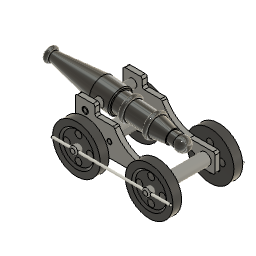
cannon v2 (Autodesk Fusion 360 design; units mm, degrees)
Autodesk Fusion 360 part; units mm, degrees
sketch "Sketch1" plane through (0, 0, 0) normal (0, 0, 1) x (1, 0, 0) in component "Component"
  line L0 (95, 0) -> (95, 20)
  line L1 (20, 50) -> (0, 50)
  line L2 (0, 50) -> (0, 0)
  line L3 (20, 50) -> (20, 40)
  line L4 (68.7228, 20) -> (95, 20)
  line L5 (75, 0) -> (75, 10)
  line L6 (75, 10) -> (20, 10)
  line L7 (20, 10) -> (20, 0)
  line L8 (0, 0) -> (20, 0)
  line L9 (75, 0) -> (95, 0)
  circle A0 centre (10, 10) radius 5
  circle A1 centre (85, 10) radius 5
  circle A2 centre (10, 40) radius 3.225
  line L10 (40, 40) -> (20, 40)
  line L11 (20, 40) -> (20, 50)
  arc A3 (40, 40) -> (71.6228, 20) centre (71.6228, 55) ccw
  arc A4 (68.7228, 20) -> (68.8018, 20.1139) centre (40, 40) ccw
  circle A5 centre (35, 24.7123) radius 2.5
  dimension "d1" = 95
  dimension "d2" = 70
  dimension "d4" = 5
  dimension "d5" = 6.45
  constraint horizontal L8
  constraint vertical L0
  constraint horizontal L1
  constraint vertical L2
  constraint coincident L2.end L8.start
  constraint vertical L3
  constraint horizontal L4
  constraint vertical L5
  constraint horizontal L6
  constraint vertical L7
  constraint collinear L8 L9
  constraint horizontal L10
  constraint vertical L11
  constraint coincident L10.start A3.start
  constraint coincident L4 A3.end
  constraint coincident A3 A4.end
  measures "d1" distance of L2.end L0.start
  measures "d2" diameter of A4
  measures "d4" diameter of A5
  measures "d5" diameter of A2
extrude "Extrude1" add sketch "Sketch1" along normal blind 5 contours L0 L1 L2 L3 L4 L5 L6 L7 L8 L9 L10 L11 A3 A4 makes body 1 in component "Component"
fillet "Fillet1" radius 2 9 edges at (95, 0, 2.5) (75, 0, 2.5) (95, 20, 2.5) (20, 0, 2.5) (0, 0, 2.5) (40, 40, 2.5) (20, 40, 2.5) (20, 50, 2.5) (0, 50, 2.5) on bodies 1 in component "Component"
fillet "Fillet2" radius 4 2 edges at (75, 10, 2.5) (20, 10, 2.5) on bodies 1 in component "Component"
copy_body "CopyPasteBodies1" bodies 1 makes body 2 in component "Component"
move_body "Move12" bodies 1 to x (1, 0, 0) y (0, 0, 1) z (0, -1, 0) at (0, -110, 0) in component "Component"
move_body "Move1" bodies 2 to x (1, 0, 0) y (0, 1, 0) z (0, 0, 1) at (0, 0, 20) in component "Component"
sketch "Sketch2" plane through (0, 0, 0) normal (0, 0, 1) x (1, 0, 0) in component "Component"
  circle A0 centre (0, 0) radius 24.5
  circle A1 centre (0, 0) radius 18
  circle A2 centre (0, 0) radius 3
  line L0 (0, 0) -> (0, 12)
  line L1 (0, 0) -> (12, 0)
  line L2 (0, 0) -> (0, -12)
  line L3 (0, 0) -> (-12, 0)
  circle A3 centre (0, 12) radius 3.5
  circle A4 centre (12, 0) radius 3.5
  circle A5 centre (0, -12) radius 3.5
  circle A6 centre (-12, 0) radius 3.5
  dimension "d12" = 49
  dimension "d13" = 36
  dimension "d14" = 6
  dimension "d15" = 12
  dimension "d16" = 12
  dimension "d17" = 12
  dimension "d18" = 12
  dimension "d19" = 7
  dimension "d20" = 7
  dimension "d21" = 7
  dimension "d22" = 7
  constraint coincident A0.centre A1.centre
  constraint concentric A0 A1
  constraint concentric A0 A2
  constraint vertical L0
  constraint perpendicular L0 L1
  constraint perpendicular L1 L2
  constraint perpendicular L2 L3
  constraint coincident L0.end A3.centre
  constraint coincident L1.end A4.centre
  constraint coincident L2.end A5.centre
  constraint coincident L3.end A6.centre
  measures "d12" diameter of A0
  measures "d13" diameter of A1
  measures "d14" diameter of A2
  measures "d15" distance of A0.centre L0.end
  measures "d16" distance of A0.centre L1.end
  measures "d17" distance of A0.centre L2.end
  measures "d18" distance of A0.centre L3.end
  measures "d19" diameter of A3
  measures "d20" diameter of A4
  measures "d21" diameter of A5
  measures "d22" diameter of A6
extrude "Extrude2" add sketch "Sketch2" against normal blind 9 separate body contours A0 | A1 makes body 3 in component "Component"
extrude "Extrude3" cut sketch "Sketch2" against normal blind 2 draft -45 contours A1 | A2 L0 L1 | A2 L1 L2 | A2 L0 L3 | A2 L2 L3 | A3 | A4 | A5 | A6 bodies 3 in component "Component"
copy_body "CopyPasteBodies2" bodies 3 makes body 4 in component "Component"
move_body "Move2" bodies 4 to x (1, 0, 0) y (0, 1, 0) z (0, 0, 1) at (0, 0, 15) in component "Component"
copy_body "CopyPasteBodies3" bodies 4 makes body 5 in component "Component"
move_body "Move3" bodies 5 to x (1, 0, 0) y (0, 1, 0) z (0, 0, 1) at (0, 0, 16) in component "Component"
copy_body "CopyPasteBodies4" bodies 4 makes body 6 in component "Component"
move_body "Move4" bodies 6 to x (1, 0, 0) y (0, 1, 0) z (0, 0, 1) at (0, 0, 30) in component "Component"
sketch "Sketch3" plane through (0, 0, 0) normal (0, 0, 1) x (1, 0, 0) in component "Component"
  circle A0 centre (0, 0) radius 3.95
  circle A1 centre (0, 0) radius 5
  circle A2 centre (0, 0) radius 6
  dimension "d27" = 7.9
  dimension "d28" = 10
  dimension "d29" = 12
  constraint coincident A0.centre A1.centre
  constraint concentric A0 A1
  constraint concentric A1 A2
  measures "d27" diameter of A0
  measures "d28" diameter of A1
  measures "d29" diameter of A2
extrude "Extrude4" add sketch "Sketch3" along normal mid plane 80 separate body contours A0 makes body 7 in component "Component"
extrude "Extrude5" add sketch "Sketch3" along normal mid plane 54 contours A1 bodies 7 in component "Component"
extrude "Extrude6" add sketch "Sketch3" along normal mid plane 44 contours A2 bodies 7 in component "Component"
sketch "Sketch4" plane through (0, 0, 0) normal (1, 0, 0) x (0, 1, 0) in component "Component"
  line L0 (0, 0) -> (0, 37.5)
  line L1 (0, 0) -> (0, -37.5)
  circle A0 centre (0, 37.5) radius 1.2
  circle A1 centre (0, -37.5) radius 1.2
  dimension "d36" = 37.5
  dimension "d37" = 37.5
  dimension "d38" = 2.4
  dimension "d39" = 2.4
  constraint coincident L0.start L1.start
  constraint vertical L0
  constraint parallel L0 L1
  constraint coincident L0.end A0.centre
  constraint coincident L1.end A1.centre
  measures "d36" distance of L0.start L0.end
  measures "d37" distance of L0.start L1.end
  measures "d38" diameter of A0
  measures "d39" diameter of A1
extrude "Extrude7" cut sketch "Sketch4" along normal mid plane 30 bodies 7 in component "Component"
fillet "Fillet3" radius 1.5 2 edges at (-3.6827, -1.4284, 40) (-3.6827, 1.4284, -40) on bodies 7 in component "Component"
copy_body "CopyPasteBodies5" bodies 7 makes body 8 in component "Component"
move_body "Move5" bodies 8 to x (1, 0, 0) y (0, 1, 0) z (0, 0, 1) at (20, 0, 0) in component "Component"
sketch "Sketch5" plane through (0, 0, 0) normal (0, 0, 1) x (1, 0, 0) in component "Component"
  circle A0 centre (0, 0) radius 2.5
  circle A1 centre (0, 0) radius 2
  dimension "d44" = 5
  dimension "d45" = 4
  constraint coincident A0.centre A1.centre
  measures "d44" diameter of A0
  measures "d45" diameter of A1
extrude "Extrude8" add sketch "Sketch5" against normal blind 54 separate body contours A0 | A1 makes body 9 in component "Component"
extrude "Extrude9" cut sketch "Sketch5" against normal blind 0.5 contours A0 | A1 bodies 9 in component "Component"
extrude "Extrude10" add sketch "Sketch5" against normal blind 0.5 draft 45 separate body contours A1 makes body 10 in component "Component"
combine "Combine1" operation add target body 10 tool bodies 9 in component "Component"
move_body "Move6" bodies 10 to x (1, 0, 0) y (0, 1, 0) z (0, 0, 1) at (0, 0, 54) in component "Component"
extrude "Extrude11" cut sketch "Sketch5" along normal blind 0.5 contours A0 | A1 bodies 10 in component "Component"
extrude "Extrude12" add sketch "Sketch5" along normal blind 0.5 draft 45 contours A1 bodies 10 in component "Component"
sketch "Sketch6" plane through (0, 0, 0) normal (0, 0, 1) x (1, 0, 0) in component "Component"
  circle A0 centre (0, 0) radius 4.25
  circle A1 centre (0, 0) radius 3.175
  dimension "d56" = 8.5
  dimension "d57" = 6.35
  constraint coincident A0.centre A1.centre
  constraint concentric A0 A1
  measures "d56" diameter of A0
  measures "d57" diameter of A1
extrude "Extrude13" add sketch "Sketch6" along normal mid plane 52 separate body contours A1 makes body 11 in component "Component"
extrude "Extrude14" add sketch "Sketch6" along normal mid plane 44 bodies 11 in component "Component"
move_body "Move7" bodies 11 to x (1, 0, 0) y (0, 1, 0) z (0, 0, 1) at (0, 0, -28) in component "Component"
move_body "Move8" bodies 11 to x (1, 0, 0) y (0, 1, 0) z (0, 0, 1) at (0, 0, 1) in component "Component"
extrude "Extrude15" add sketch "Sketch6" along normal blind 1 draft -45 contours A1 bodies 11 makes body 12 in component "Component"
move_body "Move9" bodies 12 11 to x (1, 0, 0) y (0, 1, 0) z (0, 0, 1) at (0, 0, 53) in component "Component"
extrude "Extrude16" add sketch "Sketch6" against normal blind 1 draft -45 contours A1 bodies 11 in component "Component"
move_body "Move10" bodies 12 to x (1, 0, 0) y (0, 1, 0) z (0, 0, 1) at (0, 0, -1) in component "Component"
combine "Combine2" operation add target body 11 tool bodies 12 in component "Component"
sketch "Sketch7" plane through (0, 0, 0) normal (0, 1, 0) x (1, 0, 0) in component "Component"
  line L0 (10, -10) -> (-10, -10)
  line L1 (10, -10) -> (-10, 10) construction
  line L2 (-10, -10) -> (10, 10) construction
  arc A0 (-15, -10) -> (-10, -10) centre (-12.5, -10) ccw
  arc A1 (10, -10) -> (15, -10) centre (12.5, -10) ccw
  line L3 (-15, 0) -> (15, 0)
  line L4 (15, 0) -> (22.9557, 0)
  line L5 (22.9557, -10) -> (15, -10)
  line L6 (-15, 0) -> (-30, 0)
  line L7 (-30, -6) -> (-30, -7)
  line L8 (-15, -10) -> (-30, -7)
  line L9 (-30, 0) -> (-41, 0)
  line L10 (-37, -6) -> (-30, -6)
  arc A2 (-48.2111, 0) -> (-37, -6) centre (-41, 0) ccw
  line L11 (-41, 0) -> (-48.2111, 0)
  line L12 (22.9557, 0) -> (42.9557, 0)
  line L13 (42.9557, -12.5) -> (23.9554, -12.5)
  line L14 (22.9557, -11.4996) -> (22.9557, -10)
  line L15 (22.9557, -11.4996) -> (23.9554, -12.5)
  line L16 (42.9557, 0) -> (48, 0)
  line L17 (42.9557, -12.5) -> (92.9557, -5)
  arc A3 (92.9557, -5) -> (97.956, -5) centre (95.4558, -5) ccw
  line L18 (97.956, -5) -> (97.956, -3)
  line L19 (48, 0) -> (48, -3)
  line L20 (48, -3) -> (97.956, -3)
  dimension "d66" = 2.5
  dimension "d67" = 2.5
  dimension "d72" = 12.5
  constraint horizontal L0
  constraint coincident L1 origin
  constraint coincident L2 origin
  constraint horizontal L4
  constraint horizontal L5
  constraint horizontal L6
  constraint vertical L7
  constraint horizontal L9
  constraint horizontal L10
  constraint coincident L9.end A2.centre
  constraint horizontal L12
  constraint horizontal L13
  constraint vertical L14
  constraint horizontal L16
  constraint tangent A3 L18
  constraint perpendicular L16 L19
  constraint perpendicular L18 L20
  measures "d66" distance of L0.start A1.centre
  measures "d67" distance of L0.end A0.centre
  measures "d72" distance of L12.end L13.start
revolve "Revolve1" add sketch "Sketch7" angle 360 about axis through (-15, 0, 0) along (1, 0, 0) separate body makes body 13 in component "Component"
sketch "Sketch8" plane through (0, 0, 0) normal (0, 1, 0) x (1, 0, 0) in component "Component"
  circle A0 centre (33, 0) radius 4.75
  dimension "d75" = 33
  dimension "d76" = 9.5
  measures "d75" distance of origin A0.centre
  measures "d76" diameter of A0
extrude "Extrude17" cut sketch "Sketch8" along normal mid plane 58 bodies 13 in component "Component"
move_body "Move11" bodies 13 to x (1, 0, 0) y (0, 1, 0) z (0, 0, 1) at (220, 0, 0) in component "Component"
move_body "Move13" bodies 2 to x (1, 0, 0) y (0, 0, 1) z (0, -1, 0) at (0, 90, 20) in component "Component"
move_body "Move14" bodies 3 to x (1, 0, 0) y (0, 0, 1) z (0, -1, 0) at (0, -143.5, 15.5) in component "Component"
move_body "Move15" bodies 4 to x (1, 0, 0) y (0, 0, 1) z (0, -1, 0) at (80, -148.5, 20.5) in component "Component"
move_body "Move16" bodies 5 to x (1, 0, 0) y (0, 0, 1) z (0, -1, 0) at (70, 137.5, 16.5) in component "Component"
move_body "Move17" bodies 6 to x (1, 0, 0) y (0, 0, 1) z (0, -1, 0) at (0, 171.5, 10.5) in component "Component"
move_body "Move18" bodies 7 to x (1, 0, 0) y (0, 0, -1) z (0, 1, 0) at (-40, 34, -46) in component "Component"
move_body "Move19" bodies 8 to x (1, 0, 0) y (0, 0, -1) z (0, 1, 0) at (0, 34, -46) in component "Component"
move_body "Move20" bodies 10 to x (1, 0, 0) y (0, 0, -1) z (0, 1, 0) at (30, -2.5, 17.5) in component "Component"
move_body "Move21" bodies 11 to x (1, 0, 0) y (0, 0, -1) z (0, 1, 0) at (0, -31.25, 4.75) in component "Component"
move_body "Move22" bodies 11 to x (1, 0, 0) y (0, 1, 0) z (0, 0, 1) at (0, 5, 0) in component "Component"
move_body "Move23" bodies 8 to x (1, 0, 0) y (0, 1, 0) z (0, 0, 1) at (0, -31, 0) in component "Component"
move_body "Move24" bodies 8 to x (1, 0, 0) y (0, 1, 0) z (0, 0, 1) at (65, 35, 76) in component "Component"
move_body "Move25" bodies 5 to x (1, 0, 0) y (0, 1, 0) z (0, 0, 1) at (15, -36, 13) in component "Component"
move_body "Move26" bodies 5 to x (-1, 0, 0) y (0, -1, 0) z (0, 0, 1) at (170, 141, 0.5) in component "Component"
move_body "Move27" bodies 5 to x (1, 0, 0) y (0, 1, 0) z (0, 0, 1) at (0, 9, 0) in component "Component"
move_body "Move28" bodies 7 to x (1, 0, 0) y (0, 1, 0) z (0, 0, 1) at (50, 4, 76) in component "Component"
move_body "Move29" bodies 6 to x (-1, 0, 0) y (0, -1, 0) z (0, 0, 1) at (-49, 253, 0) in component "Component"
move_body "Move30" bodies 6 to x (1, 0, 0) y (0, 1, 0) z (0, 0, 1) at (59, 0, 19) in component "Component"
move_body "Move31" bodies 6 to x (1, 0, 0) y (0, 1, 0) z (0, 0, 1) at (0, -47, 0) in component "Component"
move_body "Move32" bodies 1 to x (1, 0, 0) y (0, 1, 0) z (0, 0, 1) at (0, 121, 20) in component "Component"
move_body "Move33" bodies 3 to x (1, 0, 0) y (0, 1, 0) z (0, 0, 1) at (10, 140, 14) in component "Component"
move_body "Move34" bodies 4 to x (1, 0, 0) y (0, 1, 0) z (0, 0, 1) at (0, 160, 9) in component "Component"
move_body "Move35" bodies 4 to x (1, 0, 0) y (0, 1, 0) z (0, 0, 1) at (5, 0, 0.5) in component "Component"
move_body "Move36" bodies 10 to x (1, 0, 0) y (0, 1, 0) z (0, 0, 1) at (0, 13.5, 0) in component "Component"
move_body "Move37" bodies 1 to x (1, 0, 0) y (0, 1, 0) z (0, 0, 1) at (0, 5, 0) in component "Component"
move_body "Move38" bodies 2 to x (1, 0, 0) y (0, 1, 0) z (0, 0, 1) at (0, -5, 0) in component "Component"
move_body "Move39" bodies 3 to x (1, 0, 0) y (0, 1, 0) z (0, 0, 1) at (0, 5, 0) in component "Component"
move_body "Move40" bodies 4 to x (1, 0, 0) y (0, 1, 0) z (0, 0, 1) at (0, 5, 0) in component "Component"
move_body "Move41" bodies 5 to x (1, 0, 0) y (0, 1, 0) z (0, 0, 1) at (0, -5, 0) in component "Component"
move_body "Move42" bodies 6 to x (1, 0, 0) y (0, 1, 0) z (0, 0, 1) at (0, -5, 0) in component "Component"
move_body "Move43" bodies 10 to x (1, 0, 0) y (0, 1, 0) z (0, 0, 1) at (5, 0, 27.2) in component "Component"
move_body "Move44" bodies 11 to x (1, 0, 0) y (0, 1, 0) z (0, 0, 1) at (10, 38.25, 55.25) in component "Component"
move_body "Move45" bodies 13 to x (-1, 0, 0) y (0, 1, 0) z (0, 0, -1) at (173.5778, 38, -25) in component "Component"
move_body "Move46" bodies 13 to x (1, 0, 0) y (0, 1, 0) z (0, 0, 1) at (89.4, 0, 85) in component "Component"
move_body "Move47" bodies 13 to x (0.996195, 0, -0.087156) y (0, 1, 0) z (0.087156, 0, 0.996195) at (-4.3491, 0, -4.6109) in component "Component"
ref_plane "WorkPlane1" through (110, 0, 0) normal (1, 0, 0) x (0, 1, 0) in component "Component"
sketch "Sketch9" plane through (110, 0, 0) normal (1, 0, 0) x (0, 1, 0) in component "Component"
move_body "Move48" bodies 4 to x (1, 0, 0) y (0, 1, 0) z (0, 0, 1) at (0, 0.5, 0) in component "Component"
move_body "Move49" bodies 3 to x (1, 0, 0) y (0, 1, 0) z (0, 0, 1) at (0, 0, 0.5) in component "Component"
move_body "Move50" bodies 3 to x (1, 0, 0) y (0, 1, 0) z (0, 0, 1) at (0, 0.5, 0) in component "Component"
move_body "Move51" bodies 5 to x (1, 0, 0) y (0, 1, 0) z (0, 0, 1) at (0, -0.5, 0) in component "Component"
move_body "Move52" bodies 6 to x (1, 0, 0) y (0, 1, 0) z (0, 0, 1) at (0, -0.5, 0) in component "Component"
move_body "Move53" bodies 6 to x (1, 0, 0) y (0, 1, 0) z (0, 0, 1) at (0, 0, 0.5) in component "Component"
sketch "Sketch10" plane through (110, 0, 0) normal (1, 0, 0) x (0, 1, 0) in component "Component"
  circle A0 centre (0.5, 30) radius 1.15
  circle A1 centre (75.5, 30) radius 1.1
extrude "Extrude18" add sketch "Sketch10" against normal blind 124.5 separate body makes body 14 at (27, -0.3272, 29.2011) makes body 15 at (27, 76.4089, 30.6197) in component "Component"
move_face "OffsetFaces1" offset -0.5 2 faces at (110, 75.197, 30.2066) (110, 0.7033, 29.7451) on bodies 14 15 in component "Component"
fillet "Fillet4" radius 1.1 4 edges at (-14.5, -0.5722, 30.4159) (109.5, -0.5722, 29.5841) (-14.5, 74.4744, 30.3978) (109.5, 74.4744, 29.6022) on bodies 14 15 in component "Component"
move_body "Move54" bodies 13 to x (1, 0, 0) y (0, 1, 0) z (0, 0, 1) at (-0.8, 0, 5.7) in component "Component"
component "Component" placed x (1, 0, 0) y (0, 1, 0) z (0, 0, 1) at (0, 0, 0)
